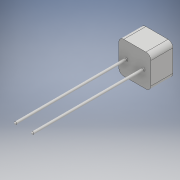
# Autodesk Inventor part: A54
Saved by Autodesk Inventor 2018 (Build 220112000, 112)
## iProperties
Created: 2020-05-16
Part Number: A54
Material: Generic
Document SubType Name: Modeling
Designer: Сергей
Density: 1 g/cm^3
Appearance: Default
Author: Сергей
Autodesk Inventor part; units mm, degrees
ref_plane "YZ Plane" through (0, 0, 0) normal (1, 0, 0) x (0, 1, 0)
ref_plane "XZ Plane" through (0, 0, 0) normal (0, 1, 0) x (-1, 0, 0)
ref_plane "XY Plane" through (0, 0, 0) normal (0, 0, 1) x (1, 0, 0)
sketch "Sketch1" plane through (0, 0, 0) normal (0, 1, 0) x (-1, 0, 0)
  line L0 (2.25, 3.25) -> (-2.25, 3.25)
  line L1 (-3.25, 2.25) -> (-3.25, -2.25)
  line L2 (-2.25, -3.25) -> (2.25, -3.25)
  line L3 (3.25, -2.25) -> (3.25, 2.25)
  line L4 (3.25, 3.25) -> (-3.25, -3.25) construction
  line L5 (-3.25, 3.25) -> (3.25, -3.25) construction
  arc A0 (-3.25, -2.25) -> (-2.25, -3.25) centre (-2.25, -2.25) ccw
  arc A1 (2.25, -3.25) -> (3.25, -2.25) centre (2.25, -2.25) ccw
  arc A2 (3.25, 2.25) -> (2.25, 3.25) centre (2.25, 2.25) ccw
  arc A3 (-2.25, 3.25) -> (-3.25, 2.25) centre (-2.25, 2.25) ccw
  point P0 (0, 0)
  dimension "d0" = 6.5
  dimension "d1" = 6.5
  dimension "d4" = 1
  constraints: 12 end point, 8 point on circle, 8 point on line, 8 tangent, 4 centre point, 3 equal radius, 2 midpoint, 2 parallel, 1 horizontal, 1 perpendicular
  measures "d0" distance of L5.end L4.end
  measures "d1" distance of L4.end L5.start
  measures "d4" radius of A0
extrude "Extrusion1" add sketch "Sketch1" along normal mid plane 4.5
sketch "Sketch4" plane through (0, 0, 0) normal (0, 0, 1) x (1, 0, 0)
  arc A0 (-1.75, -25) -> (-1.5182, -24.7516) centre (-1.7559, -24.7621) ccw
  line L0 (-1.75, -2.4144) -> (-1.75, -25)
  line L1 (-1.5182, -2.4144) -> (-1.5182, -24.7516)
  arc A1 (-1.5182, -2.4144) -> (-1.4227, -2.25) centre (-1.6226, -2.2437) ccw
  line L2 (-1.75, -2.4144) -> (-1.75, -2.25)
  line L3 (-1.75, -2.25) -> (-1.4227, -2.25)
  point P0 (0, 0)
  dimension "d27" = 0.2
  constraints: 8 end point, 4 point on circle, 2 centre point, 1 parallel
  measures "d27" radius of A1
revolve "Revolution2" add sketch "Sketch4" angle 360 about axis through (-1.75, -2.4144, 0) along (0, -1, 0)
pattern_linear "Rectangular Pattern4" count 2 spacing 3.5 along (1, 0, 0) of "Revolution2"
body "Solid1"
